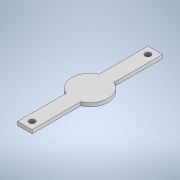
# Autodesk Inventor part: PlacaRetencion
Saved by Autodesk Inventor 2021 (Build 250183000, 183)
## iProperties
Created: 2022-11-03
Part Number: PlacaRetencion
Material: Genérico
Document SubType Name: Modeling
Designer: ivanm
Density: 1 g/cm^3
Appearance: Valor por defecto
Author: ivanm
Autodesk Inventor part; units mm, degrees
ref_plane "YZ Plane" through (0, 0, 0) normal (1, 0, 0) x (0, 1, 0)
ref_plane "XZ Plane" through (0, 0, 0) normal (0, 1, 0) x (-1, 0, 0)
ref_plane "XY Plane" through (0, 0, 0) normal (0, 0, 1) x (1, 0, 0)
sketch "Boceto1" plane through (0, 0, 0) normal (0, 1, 0) x (-1, 0, 0)
  line L0 (10, 90) -> (-10, 90)
  line L1 (-10, 90) -> (-10, -90)
  line L2 (-10, -90) -> (10, -90)
  line L3 (10, -90) -> (10, 90)
  line L4 (14, 0) -> (-14, 0) projected
  line L5 (0, -126) -> (0, 126) projected
  point P0 (0, 0)
  point P1 (10, 0)
  point P2 (0, 90)
  dimension "d0" = 20
  dimension "d1" = 180
  constraints: 8 end point, 2 midpoint, 2 parallel, 2 point on line, 1 horizontal, 1 perpendicular
  measures "d0" distance of L0.start L0.end
  measures "d1" distance of L0.end L1.end
extrude "Extrusión1" add sketch "Boceto1" along normal blind 5
sketch "Boceto2" plane through (0, 5, 0) normal (0, 1, 0) x (1, 0, 0)
  line L0 (10, 90) -> (-10, 90) projected
  line L1 (-10, 90) -> (-10, -90) projected
  line L2 (-10, -90) -> (10, -90) projected
  line L3 (10, -90) -> (10, 90) projected
  circle A0 centre (0, -80) radius 4
  circle A1 centre (0, 80) radius 4
  line L4 (0, 126) -> (0, -126) projected
  point P0 (0, 0)
  dimension "d4" = 8
  dimension "d5" = 8
  dimension "d6" = 10
  dimension "d7" = 10
  constraints: 2 centre point, 2 point on line
  measures "d4" diameter of A1
  measures "d5" diameter of A0
  measures "d6" distance from line of L2 A0.centre
  measures "d7" distance from line of L0 A1.centre
extrude "Extrusión2" cut sketch "Boceto2" against normal blind 5 contours L4 A1 | A1 L4 | L4 A0 | A0 L4
sketch "Boceto3" plane through (0, 5, 0) normal (0, 1, 0) x (1, 0, 0)
  circle A0 centre (0, 0) radius 25
  dimension "d10" = 50
  constraints: 1 centre point, 1 coincident
  measures "d10" diameter of A0
extrude "Extrusión3" add sketch "Boceto3" against normal blind 5
equation "\"d5\" = d4"
